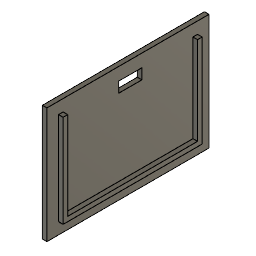
lid (Autodesk Fusion 360 design; units mm, degrees)
part number: 2026-03-23-11-12-25-279
Autodesk Fusion 360 part; units mm, degrees
sketch "Sketch11" plane through (0, 15, 0) normal (0, -1, 0) x (1, 0, 0)
  line L0 (79, 60) -> (19, 60)
  line L1 (19, 60) -> (19, 2)
  line L2 (19, 2) -> (79, 2)
  line L3 (79, 2) -> (79, 60)
  line L4 (61, 60) -> (65, 60)
  line L5 (65, 60) -> (65, 21)
  line L6 (65, 21) -> (61, 21)
  line L7 (61, 21) -> (61, 60)
  line L8 (34, 20.9953) -> (30, 20.9953)
  line L9 (30, 20.9953) -> (30, 60)
  line L10 (30, 60) -> (34, 60)
  line L11 (34, 60) -> (34, 20.9953)
  constraint horizontal L4
  constraint vertical L5
  constraint horizontal L6
  constraint vertical L7
  constraint coincident L0 L4.start
  constraint horizontal L8
  constraint vertical L9
  constraint horizontal L10
  constraint vertical L11
  constraint coincident L0 L9.end
sketch "Sketch12" plane through (0, 15, 0) normal (0, -1, 0) x (1, 0, 0)
  line L0 (65, 60) -> (65, 21)
  line L1 (65, 21) -> (61, 21)
  line L2 (61, 21) -> (61, 60)
  line L3 (61, 60) -> (34, 60)
  line L4 (34, 60) -> (34, 20.9953)
  line L5 (34, 20.9953) -> (30, 20.9953)
  line L6 (30, 20.9953) -> (30, 60)
  line L7 (30, 60) -> (19, 60)
  line L8 (19, 60) -> (19, 2)
  line L9 (19, 2) -> (79, 2)
  line L10 (79, 2) -> (79, 60)
  line L11 (79, 60) -> (65, 60)
  line L12 (61, 21) -> (34, 21)
  line L13 (34, 21) -> (34, 25)
  line L14 (34, 25) -> (61, 25)
  line L15 (61, 25) -> (61, 21)
  constraint horizontal L12
  constraint vertical L13
  constraint horizontal L14
  constraint vertical L15
  constraint coincident L4 L13.end
  constraint coincident L1.end L2.start
sketch "Sketch13" plane through (0, 0, 25) normal (0, 0, 1) x (-1, 0, 0)
  line L0 (-34, -10) -> (-61, -10)
  line L1 (-61, -15) -> (-34, -15)
  line L2 (-34, -15) -> (-34, -10)
  line L3 (-61, -10) -> (-61, -15)
sketch "Sketch14" plane through (0, 0, 25) normal (0, 0, 1) x (-1, 0, 0)
  line L0 (-34, -7) -> (-61, -7)
  line L1 (-61, -7) -> (-34, -7)
  line L2 (-34, -7) -> (-34, -10)
  line L3 (-34, -10) -> (-61, -10)
  line L4 (-61, -10) -> (-61, -7)
  line L5 (-34, -10) -> (-34, -7)
  line L6 (-61, -7) -> (-61, -10)
  line L7 (-61, -10) -> (-34, -10)
  constraint horizontal L1
  constraint vertical L2
  constraint horizontal L3
  constraint vertical L4
  constraint coincident L0.end L1.start
sketch "Sketch15" plane through (0, 0, 0) normal (0, 0, 1) x (1, 0, 0)
  line L0 (84, -30) -> (14, -30)
  line L1 (14, -30) -> (14, 20)
  line L2 (14, 20) -> (84, 20)
  line L3 (84, 20) -> (84, -30)
  line L4 (79, -25) -> (19, -25)
  line L5 (19, -25) -> (19, 15)
  line L6 (19, 15) -> (79, 15)
  line L7 (79, 15) -> (79, -25)
  line L8 (53, 10) -> (43, 10)
  line L9 (43, 10) -> (43, 14.4604)
  line L10 (43, 14.4604) -> (53, 14.4604)
  line L11 (53, 14.4604) -> (53, 10)
  line L12 (79, 15) -> (79, 20)
  line L13 (19, 15) -> (19, 20)
  dimension "d29" = 10
  constraint horizontal L0
  constraint vertical L1
  constraint horizontal L2
  constraint vertical L3
  constraint horizontal L4
  constraint vertical L5
  constraint horizontal L6
  constraint vertical L7
  constraint horizontal L8
  constraint vertical L9
  constraint horizontal L10
  constraint vertical L11
  constraint coincident L2 L12.end
  constraint perpendicular L2 L12
  constraint coincident L2 L13.end
  constraint perpendicular L2 L13
  measures "d29" distance of L8.start L8.end
sketch "Sketch16" plane through (0, 0, 0) normal (0, 0, 1) x (1, 0, 0)
  line L0 (79, -25) -> (19, -25)
  line L1 (19, -25) -> (19, 15)
  line L2 (19, 15) -> (79, 15)
  line L3 (79, 15) -> (79, -25)
  line L4 (77, -23) -> (21, -23)
  line L5 (21, -23) -> (21, 13)
  line L6 (21, 13) -> (77, 13)
  line L7 (77, 13) -> (77, -23)
  line L8 (21, 13) -> (21, 15)
  line L9 (77, 13) -> (77, 15)
  dimension "d30" = 56
  dimension "d31" = 36
  constraint horizontal L4
  constraint vertical L5
  constraint horizontal L6
  constraint vertical L7
  constraint coincident L2 L8.end
  constraint perpendicular L2 L8
  constraint coincident L2 L9.end
  constraint perpendicular L2 L9
  measures "d30" distance of L4.start L4.end
  measures "d31" distance of L4.start L6.end
extrude "Extrude10" add sketch "Sketch15" sketch "Sketch16" against normal blind 4 contours L0 L1 L2 L3 L4 L5 L7 L12 L13 | L2 L6 L12 L13 of sketch 2 contours L4 L5 L6 L7 makes body 1 at (59, -28.3333, 0) makes body 2 at (39.6667, -11, 0)
extrude "Extrude11" add sketch "Sketch16" against normal blind 4 separate body contours L2 L6 L8 L9 makes body 3
extrude "Extrude12" add sketch "Sketch16" against normal blind 2 separate body contours L0 L1 L2 L3 L4 L5 L7 L8 L9 makes body 4
move_body "Move7" bodies 1 4 2 3 to x (1, 0, 0) y (0, 1, 0) z (0, 0, 1) at (0, 0, -5)
extrude "Extrude13" cut 3 faces at (59, -28.3333, -9) (39.6667, -11, -9) (39.6667, 14.3333, -9) along direction (0, 0, 1) blind 2 on bodies 1 2 3 bodies 1 2 3
extrude "Extrude14" add 1 faces at (39.6667, -24.3333, -7) along direction (0, 0, -1) blind 2 on bodies 4 bodies 1 4 2 3
sketch "Sketch17" plane through (0, 0, -7) normal (0, 0, -1) x (1, 0, 0)
  line L0 (21, 23) -> (21, -15)
  line L1 (21, -15) -> (19, -15)
  line L2 (19, -15) -> (19, 25)
  line L3 (19, 25) -> (79, 25)
  line L4 (79, 25) -> (79, -15)
  line L5 (79, -15) -> (77, -15)
  line L6 (77, -15) -> (77, 23)
  line L7 (77, 23) -> (21, 23)
  line L8 (14, -20) -> (84, -20)
  line L9 (84, -20) -> (84, 30)
  line L10 (84, 30) -> (14, 30)
  line L11 (14, 30) -> (14, -20)
  line L12 (43, -10) -> (53, -10)
  line L13 (53, -10) -> (53, -14.5)
  line L14 (53, -14.5) -> (43, -14.5)
  line L15 (43, -14.5) -> (43, -10)
  line L16 (43, -10) -> (53, -10)
  line L17 (53, -10) -> (53, -14.5)
  line L18 (53, -14.5) -> (43, -14.5)
  line L19 (43, -14.5) -> (43, -10)
  constraint horizontal L12
  constraint vertical L13
  constraint horizontal L14
  constraint vertical L15
  constraint horizontal L16
  constraint vertical L17
  constraint horizontal L18
  constraint vertical L19
extrude "Extrude15" cut sketch "Sketch17" against normal blind 4 contours L12 L13 L14 L15 L16 L17 L18 L19 bodies 1
move_body "Move8" bodies 1 to x (0, -1, 0) y (0, 0, 1) z (-1, 0, 0) at (-55, 154, 21)
move_body "Move9" bodies 1 to x (1, 0, 0) y (0, 1, 0) z (0, 0, 1) at (0, -90, 0)
